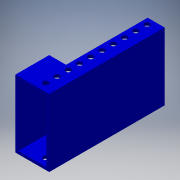
# Autodesk Inventor part: 2018 Scissor Stand Off Outside B
Saved by Autodesk Inventor 2018 (Build 220112000, 112)
## iProperties
Created: 2018-01-26
Part Number: 2018 Scissor Stand Off Outside B
Material: Generic
Document SubType Name: Modeling
Designer: Apple
Density: 1 g/cm^3
Appearance: Default
Author: Apple
Autodesk Inventor part; units mm, degrees
ref_plane "YZ Plane" through (0, 0, 0) normal (1, 0, 0) x (0, 1, 0)
ref_plane "XZ Plane" through (0, 0, 0) normal (0, 1, 0) x (-1, 0, 0)
ref_plane "XY Plane" through (0, 0, 0) normal (0, 0, 1) x (1, 0, 0)
sketch "Sketch1" plane through (0, 0, 0) normal (0, 0, 1) x (1, 0, 0)
  line L0 (20.1195, -38.0715) -> (-17.9805, -38.0715)
  line L1 (-17.9805, -38.0715) -> (-17.9805, -114.2715)
  line L2 (-17.9805, -114.2715) -> (20.1195, -114.2715)
  line L3 (20.1195, -114.2715) -> (20.1195, -38.0715)
  line L4 (16.9445, -111.0965) -> (-14.8055, -111.0965)
  line L5 (-14.8055, -111.0965) -> (-14.8055, -41.2465)
  line L6 (-14.8055, -41.2465) -> (16.9445, -41.2465)
  line L7 (16.9445, -41.2465) -> (16.9445, -111.0965)
  point P0 (0, 0)
  dimension "d0" = 76.2
  dimension "d1" = 38.1
  dimension "d2" = 3.175
  constraints: 16 end point, 4 parallel, 2 perpendicular, 1 horizontal, 3 other
  measures "d0" distance of L0.end L1.end
  measures "d1" distance of L1.end L2.end
  measures "d2" distance between parallel lines of L2 L4
extrude "Extrusion1" add sketch "Sketch1" along normal blind 130.175
sketch "Sketch2" plane through (-17.9805, -114.2715, 0) normal (-1, 0, 0) x (0, 0, 1)
  line L0 (0, 76.2) -> (130.175, 76.2) projected
  line L1 (0, 76.2) -> (0, 0) projected
  line L2 (0, 0) -> (130.175, 0) projected
  line L3 (130.175, 76.2) -> (130.175, 0) projected
  line L4 (0, 76.2) -> (92.075, 76.2)
  line L5 (92.075, 76.2) -> (92.075, 38.1)
  line L6 (92.075, 38.1) -> (0, 38.1)
  line L7 (0, 38.1) -> (0, 76.2)
  point P0 (0, 114.2715)
  dimension "d27" = 38.1
  dimension "d28" = 38.1
  constraints: 8 end point, 2 parallel, 1 horizontal, 1 perpendicular
  measures "d27" distance between parallel lines of L2 L6
  measures "d28" distance between parallel lines of L5 L3
extrude "Extrusion2" cut sketch "Sketch2" against normal blind 19.05 contours L0 L5 L6 L1
sketch "Sketch3" plane through (-17.9805, -114.2715, 0) normal (0, -1, 0) x (1, 0, 0)
  line L0 (38.1, 0) -> (38.1, 130.175) projected
  line L1 (0, 130.175) -> (38.1, 130.175) projected
  point P0 (17.9805, 0)
  point P1 (25.4, 121.285)
  point P2 (25.4, 108.585)
  point P3 (25.4, 95.885)
  point P4 (25.4, 83.185)
  point P5 (25.4, 70.485)
  point P6 (25.4, 57.785)
  point P7 (25.4, 45.085)
  point P8 (25.4, 32.385)
  point P9 (25.4, 19.685)
  point P10 (25.4, 6.985)
  dimension "d9" = 12.7
  dimension "d10" = 8.89
  dimension "d13" = 12.7
  constraints: 1 vertical, 9 other
  measures "d9" distance from line of point (25.4, 121.285) L0
  measures "d10" distance from line of L1 point (25.4, 121.285)
  measures "d13" distance of point (25.4, 121.285) point (25.4, 108.585)
hole "Hole1" at (7.4195, -114.2715, 121.285) at (7.4195, -114.2715, 108.585) at (7.4195, -114.2715, 95.885) at (7.4195, -114.2715, 83.185) at (7.4195, -114.2715, 70.485) at (7.4195, -114.2715, 57.785) at (7.4195, -114.2715, 45.085) at (7.4195, -114.2715, 32.385) at (7.4195, -114.2715, 19.685) at (7.4195, -114.2715, 6.985) direction (0, 1, 0) diameter 6.35 end through all
body "Solid1"
